Autodesk Fusion 360 part; units mm, degrees
(part 2 of 2)
fillet "圆角4" radius 4 1 edges at (32.5, 0, -4) on bodies 1
fillet "圆角5" radius 4 1 edges at (0, 20.105, -2) on bodies 1
fillet "圆角6" radius 4 1 edges at (65, 20.105, -2) on bodies 1
delete_face "删除面1" 1 faces at (21.6667, 3.8097, -3.9955) on bodies 1
ref_plane "工作平面1" through (32.5, 0, -4) normal (0, -0.087156, 0.996195) x (1, 0, 0)
sketch "草图8" plane through (0, 0.3473, -3.9696) normal (0, -0.087156, 0.996195) x (1, 0, 0)
  line L0 (0, -0.3486) -> (65, -0.3486)
  line L1 (0, -0.3486) -> (0, -30.3486)
  line L2 (0, -30.3486) -> (65, -30.3486)
  line L3 (65, -30.3486) -> (65, -0.3486)
  line L4 (0, -15.3486) -> (65, -15.3486) construction
  circle A0 centre (12.5, -15.3486) radius 2.15
  line L5 (32.5, -0.3486) -> (32.5, -30.3486) construction
  circle A1 centre (52.5, -15.3486) radius 2.15
  point P0 (0, -0.3486)
  point P1 (65, -0.3486)
  dimension "d62" = 30
  dimension "d64" = 4.3
  dimension "d65" = 40
  constraint horizontal L0
  constraint coincident P0 L0.start
  constraint coincident P1 L0.end
  constraint perpendicular L0 L1
  constraint perpendicular L1 L2
  constraint perpendicular L2 L3
  constraint midpoint L1 L4.start
  constraint midpoint L3 L4.end
  constraint coincident L4 A0.centre
  constraint midpoint L0 L5.start
  constraint midpoint L2 L5.end
  constraint coincident L4 A1.centre
  constraint symmetric A0 L5 A1
  measures "d62" distance of P0 L1.end
  measures "d64" diameter of A0
  measures "d65" distance of A0.centre A1.centre
extrude "拉伸9" add sketch "草图8" along normal blind 4 separate body makes body 2
extrude "拉伸10" add 1 faces at (21.6667, -0.2324, -1.3435) along direction (0, 0.996195, 0.087156) blind 0.877 on bodies 2 bodies 1 2
fillet "圆角7" radius 4 2 edges at (65, -30.0602, -4.6223) (0, -30.0602, -4.6223) on bodies 1
fillet "圆角8" radius 4 1 edges at (32.5, 0, 0.0153) on bodies 1
delete_face "删除面2" 1 faces at (43.3333, -3.2596, -0.2503) on bodies 1
delete_face "删除面3" 1 faces at (21.6667, 4.4199, 0.1854) on bodies 1
extrude "拉伸3" [suppressed]
sketch "草图4" plane through (0, 0, 0) normal (0, 1, 0) x (1, 0, 0)
  line L0 (0, 0) -> (65, 0)
  line L1 (65, 0) -> (65, -25.17)
  line L2 (65, -25.17) -> (0, -25.17)
  line L3 (0, -25.17) -> (0, 0)
  line L4 (0, -7) -> (65, -7) construction
  circle A0 centre (10, -7) radius 1.25
  line L5 (32.5, 0) -> (32.5, -25.17) construction
  circle A1 centre (55, -7) radius 1.25
  line L6 (0, -21.17) -> (65, -21.17)
  dimension "d23" = 25.17
  dimension "d24" = 65
  dimension "d25" = 2.5
  dimension "d26" = 45
  dimension "d27" = 7
  dimension "d28" = 4
  constraint horizontal L0
  constraint vertical L1
  constraint horizontal L2
  constraint vertical L3
  constraint coincident L0.start L3.end
  constraint coincident L4 A0.centre
  constraint midpoint L0 L5.start
  constraint midpoint L2 L5.end
  constraint symmetric A0 L5 A1
  constraint coincident L3 L4.start
  constraint coincident L1 L4.end
  constraint coincident L3 L6.start
  constraint coincident L1 L6.end
  constraint perpendicular L1 L6
  measures "d23" distance of L0.start L2.end
  measures "d24" distance of L0.start L0.end
  measures "d25" diameter of A0
  measures "d26" distance of A0.centre A1.centre
  measures "d27" distance of L0 L4
  measures "d28" distance of L2.end L6.start
extrude "拉伸4" [suppressed]
sketch "草图5" plane through (0, 0, 25.17) normal (0, 0, 1) x (1, 0, 0)
  line L0 (0, 0) -> (65, 0)
  line L1 (65, 0) -> (65, 4)
  line L2 (65, 4) -> (0, 4)
  line L3 (0, 4) -> (0, 0)
equation "d23 = 14 mm + 7.17 mm + 4 mm"
equation "d39 = 16.105 mm + 4 mm"
